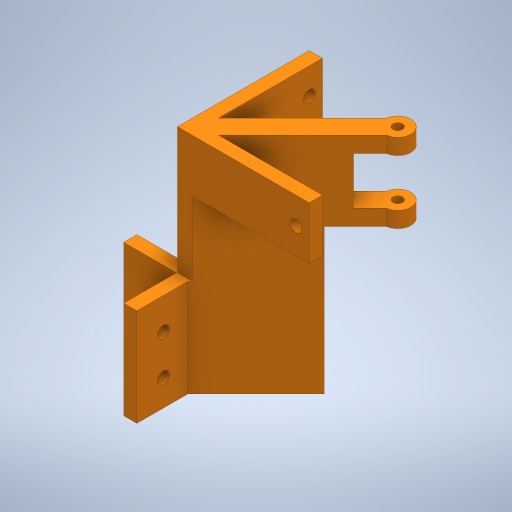
# Autodesk Inventor part: PulleyHolderXY
Saved by Autodesk Inventor 2023 (Build 270158000, 158)
## iProperties
Created: 2022-09-02
Part Number: PulleyHolderXY
Material: PET Plastic
Document SubType Name: Modeling
Designer: Nathann
Density: 1.541 g/cm^3
Appearance: Orange
Author: Nathann
Autodesk Inventor part; units mm, degrees
ref_plane "YZ Plane" through (0, 0, 0) normal (1, 0, 0) x (0, 1, 0)
ref_plane "XZ Plane" through (0, 0, 0) normal (0, 1, 0) x (-1, 0, 0)
sketch "Sketch1" plane through (0, 0, 0) normal (0, 0, 1) x (1, 0, 0)
  line L0 (-9.7719, -3.7131) -> (-29.115, -3.7131)
  line L1 (-29.115, -3.7131) -> (-29.115, -8.7131)
  line L2 (-29.115, -8.7131) -> (-9.115, -8.7131)
  line L3 (-9.115, -8.7131) -> (-9.115, -28.7131)
  line L4 (-9.115, -28.7131) -> (-4.115, -28.7131)
  line L5 (-4.115, -28.7131) -> (-4.115, -9.37)
  line L6 (-9.7719, -3.7131) -> (27.9352, 33.994)
  line L7 (33.5921, 28.3372) -> (-4.115, -9.37)
  circle A0 centre (32.885, 33.2869) radius 1.85
  arc A1 (33.5921, 28.3372) -> (27.9352, 33.994) centre (32.885, 33.2869) ccw
  dimension "d0" = 20
  dimension "d1" = 20
  dimension "d2" = 5
  dimension "d3" = 5
  dimension "d7" = 42
  dimension "d8" = 42
  dimension "d9" = 3.7
  dimension "d18" = 5
  dimension "d19" = 135
  dimension "d67" = 8
  constraints: 16 end point, 4 parallel, 2 centre point, 2 perpendicular, 2 point on circle, 1 coincident, 1 horizontal
  measures "d0" distance from line of L1.end L3
  measures "d1" distance between parallel lines of L4 L2
  measures "d2" distance of L0.end L1.end
  measures "d3" distance of L3.end L4.end
  measures "d7" distance from line of A0.centre L2
  measures "d8" distance from line of L3 A0.centre
  measures "d9" diameter of A0
  measures "d18" radius of A1
  measures "d19" angle of L7 L5
  measures "d67" distance between parallel lines of L7 L6
extrude "Extrusion1" add sketch "Sketch1" along normal blind 30
ref_plane "Work Plane1" through (0, 0, 24) normal (0, 0, 1) x (1, 0, 0)
sketch "Sketch3" plane through (0, 0, 24) normal (0, 0, 1) x (1, 0, 0)
  circle A0 centre (32.885, 33.2869) radius 1.85 projected
  circle A1 centre (32.885, 33.2869) radius 12.5
  point P0 (0, 0)
  dimension "d13" = 25
  constraints: 1 centre point, 1 coincident
  measures "d13" diameter of A1
extrude "Extrusion3" cut sketch "Sketch3" against normal blind 18
sketch "Sketch5" plane through (0, 0, 0) normal (0, 0, -1) x (-1, 0, 0)
  circle A0 centre (-32.885, 33.2869) radius 1.85 projected
  line L0 (29.115, -8.7131) -> (29.115, -3.7131) projected
  line L1 (29.115, -3.7131) -> (9.7719, -3.7131) projected
  line L2 (9.7719, -3.7131) -> (-27.9352, 33.994) projected
  arc A1 (-27.9352, 33.994) -> (-33.5921, 28.3372) centre (-32.885, 33.2869) ccw projected
  line L3 (-33.5921, 28.3372) -> (4.115, -9.37) projected
  line L4 (4.115, -9.37) -> (4.115, -28.7131) projected
  line L5 (4.115, -28.7131) -> (9.115, -28.7131) projected
  line L6 (9.115, -28.7131) -> (9.115, -8.7131) projected
  line L7 (9.115, -8.7131) -> (29.115, -8.7131) projected
  line L8 (4.115, -9.37) -> (9.7719, -3.7131)
  point P0 (0, 0)
  constraints: 2 end point
extrude "Extrusion5" add sketch "Sketch5" along normal blind 55
sketch "Sketch8" plane through (-9.115, -28.7131, -55) normal (-1, 0, 0) x (0, 0, 1)
  circle A0 centre (10, 10) radius 2.25
  line L0 (85, 0) -> (0, 0) projected
  line L1 (0, 0) -> (0, 20) projected
  circle A1 centre (25, 10) radius 2.25
  point P0 (55, 28.7131)
  dimension "d40" = 4.5
  dimension "d41" = 10
  dimension "d42" = 10
  dimension "d43" = 4.5
  dimension "d44" = 10
  dimension "d45" = 15
  constraints: 2 centre point
  measures "d40" diameter of A0
  measures "d41" distance from line of L0 A0.centre
  measures "d42" distance from line of L1 A0.centre
  measures "d43" diameter of A1
  measures "d44" distance from line of L0 A1.centre
  measures "d45" distance of A0.centre A1.centre
sketch "Sketch9" plane through (-29.115, -3.7131, 30) normal (0, 1, 0) x (1, 0, 0)
  circle A0 centre (10, 75) radius 2.25
  circle A1 centre (10, 60) radius 2.25
  line L0 (0, 85) -> (19.3431, 85) projected
  line L1 (0, 0) -> (0, 85) projected
  point P0 (29.115, 30)
  dimension "d46" = 10
  dimension "d47" = 10
  dimension "d48" = 10
  dimension "d49" = 15
  dimension "d50" = 4.5
  dimension "d51" = 4.5
  constraints: 2 centre point
  measures "d46" distance from line of L0 A0.centre
  measures "d47" distance from line of L1 A0.centre
  measures "d48" distance from line of L1 A1.centre
  measures "d49" distance of A0.centre A1.centre
  measures "d50" diameter of A0
  measures "d51" diameter of A1
extrude "Extrusion8" cut sketch "Sketch9" against normal mid plane 20
extrude "Extrusion9" cut sketch "Sketch8" against normal blind 20
sketch "Sketch10" plane through (0, 0, 30) normal (0, 0, 1) x (1, 0, 0)
  line L0 (-10.9341, 2.1461) -> (2.7686, -11.5566)
  line L1 (2.7686, -11.5566) -> (2.7686, -32.7748)
  line L2 (2.7686, -32.7748) -> (-29.9337, -32.7748)
  line L3 (-29.9337, -32.7748) -> (-29.9337, 2.1461)
  line L4 (-29.9337, 2.1461) -> (-10.9341, 2.1461)
  line L5 (-8.915, -8.5131) -> (-0.2749, -8.5131)
  line L6 (-8.915, -8.5131) -> (-8.915, 0.127)
  line L7 (-9.115, -8.7131) -> (-9.115, -28.7131) projected
  point P0 (0, 0)
  point P1 (-4.0828, -4.7053)
  dimension "d56" = 135
  dimension "d65" = 0.2
  dimension "d66" = 0.2
  constraints: 14 end point, 4 perpendicular, 2 point on line, 1 horizontal, 1 midpoint, 1 vertical
  measures "d56" angle of L0 L4
  measures "d65" distance between parallel lines of L6 L7
  measures "d66" distance from line of L7.start L5
extrude "Extrusion10" cut sketch "Sketch10" against normal blind 48 contours L0 L6 L5 L1 L2 L3 L4
sketch "Sketch12" plane through (0, 0, 30) normal (0, 0, 1) x (1, 0, 0)
  line L0 (-8.915, -8.5131) -> (-3.2582, -8.5131) projected
  line L1 (-3.2582, -8.5131) -> (-8.915, -8.5131)
  line L2 (-8.915, -8.5131) -> (-8.915, 41.4826)
  line L3 (-8.915, 41.4826) -> (-3.915, 41.4826)
  line L4 (-8.915, -2.8562) -> (-8.915, -8.5131) projected
  line L5 (-8.915, -8.5131) -> (41.085, -8.5131)
  line L6 (41.085, -8.5131) -> (41.085, -3.5131)
  line L7 (41.085, -3.5131) -> (-8.915, -3.5131)
  line L8 (-8.915, -3.5131) -> (-8.915, -8.5131)
  line L9 (-3.915, -8.5131) -> (-3.915, 41.4826)
  point P0 (0, 0)
  point P1 (-8.915, -3.5131)
  point P2 (-3.915, -3.5131)
  dimension "d68" = 5
  dimension "d70" = 50
  dimension "d71" = 50
  dimension "d75" = 0
  dimension "d76" = 5
  constraints: 16 end point, 4 parallel, 2 horizontal, 2 perpendicular, 1 point on line
  measures "d68" distance of L5.end L6.end
  measures "d70" distance of L3.end L0.end
  measures "d71" distance of L6.end L7.end
  measures "d75" distance between parallel lines of L4 L2
  measures "d76" distance between parallel lines of L9 L2
extrude "Extrusion12" add sketch "Sketch12" against normal blind 20
sketch "Sketch13" plane through (-3.915, 2.1438, 30) normal (1, 0, 0) x (0, 0, -1)
  circle A0 centre (10, 34.3388) radius 2.25
  line L0 (0, 0) -> (0, 39.3388) projected
  line L1 (0, 39.3388) -> (20, 39.3388) projected
  point P0 (30, -2.1438)
  dimension "d77" = 10
  dimension "d78" = 5
  dimension "d79" = 4.5
  constraints: 1 centre point
  measures "d77" distance from line of L0 A0.centre
  measures "d78" distance from line of L1 A0.centre
  measures "d79" diameter of A0
sketch "Sketch14" plane through (1.7418, -3.5131, 30) normal (0, 1, 0) x (1, 0, 0)
  circle A0 centre (34.3431, 10) radius 2.25
  line L0 (39.3431, 0) -> (39.3431, 20) projected
  line L1 (39.3431, 0) -> (0, 0) projected
  point P0 (-1.7418, 30)
  dimension "d80" = 5
  dimension "d81" = 4.5
  dimension "d82" = 10
  constraints: 1 centre point
  measures "d80" distance from line of L0 A0.centre
  measures "d81" diameter of A0
  measures "d82" distance from line of L1 A0.centre
extrude "Extrusion13" cut sketch "Sketch13" against normal blind 20
extrude "Extrusion14" cut sketch "Sketch14" against normal blind 20
sketch "Sketch15" plane through (0, 0, -55) normal (0, 0, -1) x (-1, 0, 0)
  line L0 (-27.9352, 33.994) -> (3.915, 2.1438) projected
  line L1 (-16.0867, 22.1455) -> (-21.7436, 16.4887)
  line L2 (-1.7418, -3.5131) -> (-33.5921, 28.3372) projected
  line L3 (-24.5175, 13.7148) -> (-29.4962, 12.412)
  circle A0 centre (-32.885, 33.2869) radius 1.85 projected
  line L4 (29.115, -8.7131) -> (29.115, -3.7131) projected
  line L5 (29.115, -3.7131) -> (9.7719, -3.7131) projected
  line L6 (9.7719, -3.7131) -> (-27.9352, 33.994) projected
  arc A1 (-27.9352, 33.994) -> (-33.5921, 28.3372) centre (-32.885, 33.2869) ccw projected
  line L7 (-33.5921, 28.3372) -> (4.115, -9.37) projected
  line L8 (4.115, -9.37) -> (4.115, -28.7131) projected
  line L9 (4.115, -28.7131) -> (9.115, -28.7131) projected
  line L10 (9.115, -28.7131) -> (9.115, -8.7131) projected
  line L11 (9.115, -8.7131) -> (29.115, -8.7131) projected
  point P0 (0, 0)
  constraints: 4 end point, 3 point on line
extrude "Extrusion15" cut sketch "Sketch15" against normal blind 55 contours L0 L1 L2 A1
equation "\"d8\" = d7"
equation "\"d43\" = d40"
equation "\"d44\" = d41"
equation "\"d71\" = d70"
equation "\"RodDiameter\" = 8"
equation "\"VerticalBearingOD\" = 16"
equation "\"PrintingClearance\" = 0.2"
equation "\"TubeID\" = 18"
equation "\"XLinearBearingOD\" = 19"
body "Solid1"
